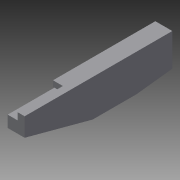
# Autodesk Inventor part: FrontSkidRight
Saved by Autodesk Inventor 2014 (Build 180170000, 170)
## iProperties
Created: 2016-02-03
Part Number: FrontSkidRight
Material: Generic
Document SubType Name: Modeling
Designer: zoldberg
Density: 1 g/cm^3
Appearance: Default
Author: zoldberg
Autodesk Inventor part; units mm, degrees
ref_plane "YZ Plane" through (0, 0, 0) normal (1, 0, 0) x (0, 1, 0)
ref_plane "XZ Plane" through (0, 0, 0) normal (0, 1, 0) x (-1, 0, 0)
ref_plane "XY Plane" through (0, 0, 0) normal (0, 0, 1) x (1, 0, 0)
sketch "Sketch1" plane through (0, 0, 0) normal (0, 0, 1) x (1, 0, 0)
  line L0 (19.05, -44.45) -> (-19.05, -44.45)
  line L1 (-19.05, -44.45) -> (-19.05, 44.45)
  line L2 (-19.05, 44.45) -> (19.05, 44.45)
  line L3 (19.05, 44.45) -> (19.05, -44.45)
  line L4 (19.05, -44.45) -> (-19.05, 44.45) construction
  line L5 (-19.05, -44.45) -> (19.05, 44.45) construction
  point P0 (0, 0)
  dimension "d0" = 38.1
  dimension "d1" = 88.9
  constraints: 12 end point, 2 midpoint, 2 parallel, 1 horizontal, 1 perpendicular
  measures "d0" distance of L1.end L2.end
  measures "d1" distance of L0.end L1.end
extrude "Extrusion1" add sketch "Sketch1" along normal blind 673.8874
sketch "Sketch2" plane through (0, 0, 673.8874) normal (0, 0, 1) x (1, 0, 0)
  line L0 (19.05, -44.45) -> (19.05, 44.45) projected
  line L1 (19.05, 44.45) -> (-19.05, 44.45) projected
  line L2 (19.05, 31.75) -> (3.175, 31.75)
  line L3 (3.175, 31.75) -> (3.175, 28.575)
  line L4 (3.175, 28.575) -> (19.05, 28.575)
  line L5 (19.05, 28.575) -> (19.05, 31.75)
  line L6 (-19.05, 44.45) -> (-19.05, -44.45) projected
  line L7 (0, 25.0075) -> (0, 34.7359)
  line L8 (-19.05, 31.75) -> (-3.175, 31.75)
  line L9 (-3.175, 31.75) -> (-3.175, 28.575)
  line L10 (-3.175, 28.575) -> (-19.05, 28.575)
  line L11 (-19.05, 28.575) -> (-19.05, 31.75)
  point P0 (0, 0)
  dimension "d4" = 12.7
  dimension "d5" = 3.175
  dimension "d6" = 15.875
  constraints: 18 end point, 4 symmetric about line, 3 parallel, 1 horizontal, 1 perpendicular, 1 point on line
  measures "d4" distance between parallel lines of L2 L1
  measures "d5" distance of L2.end L3.end
  measures "d6" distance of L3.end L4.end
sketch "Sketch4" plane through (19.05, -44.45, 673.8874) normal (1, 0, 0) x (0, 0, -1)
  line L0 (0, 0) -> (0, 88.9) projected
  line L1 (673.8874, 0) -> (0, 0) projected
  line L2 (673.8874, 88.9) -> (673.8874, 0) projected
  line L3 (673.8874, 6.35) -> (0, 6.35)
  line L4 (152.4, 6.35) -> (0, 47.1855)
  line L5 (250.444, 6.35) -> (421.8705, 26.67)
  line L6 (421.8705, 26.67) -> (673.8874, 26.67)
  point P0 (673.8874, 73.025)
  point P1 (0, 73.025)
  point P2 (673.8874, 44.45)
  dimension "d15" = 6.35
  dimension "d20" = 152.4
  dimension "d21" = 165
  dimension "d23" = 20.32
  dimension "d24" = 98.044
  dimension "d25" = 173.24
  constraints: 8 end point, 6 point on line, 2 perpendicular
  measures "d15" distance between parallel lines of L1 L3
  measures "d20" distance of L4.start L3.end
  measures "d21" angle of L3 L4
  measures "d23" distance between parallel lines of L3 L6
  measures "d24" distance of L4.start L5.start
  measures "d25" angle of L5 L3
extrude "Extrusion3" cut sketch "Sketch4" against normal blind 152.4
sketch "Sketch5" plane through (-19.05, 44.45, 0) normal (0, 1, 0) x (1, 0, 0)
  line L0 (38.1, -673.8874) -> (15.875, -673.8874)
  line L1 (15.875, -673.8874) -> (15.875, -572.2874)
  line L2 (15.875, -572.2874) -> (38.1, -572.2874)
  line L3 (38.1, -572.2874) -> (38.1, -673.8874)
  line L4 (19.05, -558.0239) -> (19.05, -615.4069)
  line L5 (0, -673.8874) -> (22.225, -673.8874)
  line L6 (22.225, -673.8874) -> (22.225, -572.2874)
  line L7 (22.225, -572.2874) -> (0, -572.2874)
  line L8 (0, -572.2874) -> (0, -673.8874)
  point P0 (19.05, 0)
  dimension "d28" = 22.225
  dimension "d29" = 101.6
  constraints: 18 end point, 3 parallel, 3 symmetric about line, 1 horizontal, 1 perpendicular
  measures "d28" distance of L1.end L2.end
  measures "d29" distance of L0.end L1.end
extrude "Extrusion4" cut sketch "Sketch5" against normal blind 15.875 contours L0 L1 L2 L6 | L5 L8 L7 L1
sketch "Sketch6" plane through (-19.05, 44.45, 0) normal (0, 1, 0) x (1, 0, 0)
  line L0 (38.1, 0) -> (38.1, -673.8874) projected
  line L1 (0, 0) -> (38.1, 0) projected
  line L2 (38.1, -215.9) -> (0, -215.9)
  line L3 (0, -215.9) -> (0, -342.9)
  line L4 (0, -342.9) -> (38.1, -342.9)
  line L5 (38.1, -342.9) -> (38.1, -215.9)
  point P0 (38.1, -572.2874)
  point P1 (19.05, 0)
  dimension "d32" = 127
  dimension "d33" = 215.9
  dimension "d36" = 38.1
  constraints: 8 end point, 2 parallel, 1 horizontal, 1 perpendicular, 1 point on line
  measures "d32" distance of L3.end L2.end
  measures "d33" distance between parallel lines of L1 L2
  measures "d36" distance of L2.start L2.end
extrude "Extrusion5" cut sketch "Sketch6" against normal blind 15.875
sketch "Sketch7" plane through (0, 0, 0) normal (0, 0, -1) x (-1, 0, 0)
  line L0 (41.2519, 59.9443) -> (-67.5031, 59.9443)
  line L1 (-67.5031, 59.9443) -> (-67.5031, -55.7754)
  line L2 (-67.5031, -55.7754) -> (41.2519, -55.7754)
  line L3 (41.2519, -55.7754) -> (41.2519, 59.9443)
  point P0 (0, 0)
  constraints: 8 end point, 2 parallel, 1 horizontal, 1 perpendicular
extrude "Extrusion6" cut sketch "Sketch7" against normal blind 342.9
extrude "Extrusion7" cut sketch "Sketch2" against normal blind 508 contours L8 L9 L10 L6
body "Solid1"
